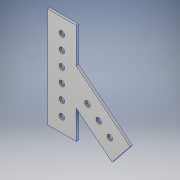
# Autodesk Inventor part: SUP_011_Top4BarBarGusset
Saved by Autodesk Inventor 2018.3 (Build 223284000, 284)
## iProperties
Created: 2020-02-09
Part Number: SUP_011_Top4BarBarGusset
Material: Aluminum 6061
Document SubType Name: Modeling
Designer: 22barlalex
Density: 2.7 g/cm^3
Appearance: Aluminum - Flat
Author: 22barlalex
Autodesk Inventor part; units mm, degrees
ref_plane "YZ Plane" through (0, 0, 0) normal (1, 0, 0) x (0, 1, 0)
ref_plane "XZ Plane" through (0, 0, 0) normal (0, 1, 0) x (-1, 0, 0)
ref_plane "XY Plane" through (0, 0, 0) normal (0, 0, 1) x (1, 0, 0)
sketch "Sketch1" plane through (0, 0, 0) normal (0, 0, 1) x (1, 0, 0)
  line L0 (0, 0) -> (0, 88.9)
  line L1 (0, 88.9) -> (25.4, 88.9)
  line L2 (25.4, 88.9) -> (25.4, 57.9416)
  line L3 (25.4, 57.9416) -> (72.9934, 19.8257)
  line L4 (72.9934, 19.8257) -> (57.1157, 0)
  line L5 (57.1157, 0) -> (25.4, 25.4)
  line L6 (25.4, 25.4) -> (25.4, 0)
  line L7 (25.4, 0) -> (0, 0)
  dimension "d0" = 25.4
  dimension "d1" = 25.4
  dimension "d3" = 25.4
  dimension "d5" = 51.31
  dimension "d18" = 88.9
  constraints: 16 end point, 4 perpendicular, 3 point on line, 1 parallel, 1 vertical
  measures "d0" distance between parallel lines of L3 L5
  measures "d1" distance between parallel lines of L0 L6
  measures "d3" distance of L6.end L5.end
  measures "d5" angle of L5 L6
  measures "d18" distance between parallel lines of L1 L7
extrude "Extrusion1" add sketch "Sketch1" along normal blind 2.032
sketch "Sketch3" plane through (0, 0, 2.032) normal (0, 0, 1) x (1, 0, 0)
  line L0 (25.4, 57.9416) -> (25.4, 88.9) projected
  line L1 (0, 0) -> (25.4, 0) projected
  line L2 (72.9934, 19.8257) -> (25.4, 57.9416) projected
  line L3 (57.1157, 0) -> (72.9934, 19.8257) projected
  point P0 (12.7, 12.7)
  point P1 (12.7, 25.4)
  point P2 (12.7, 38.1)
  point P3 (12.7, 50.8)
  point P4 (12.7, 63.5)
  point P5 (12.7, 76.2)
  point P6 (55.1417, 17.8517)
  point P7 (45.2289, 25.7906)
  point P8 (35.316, 33.7294)
  dimension "d8" = 12.7
  dimension "d9" = 12.7
  dimension "d10" = 12.7
  dimension "d11" = 12.7
  dimension "d12" = 12.7
  dimension "d13" = 12.7
  dimension "d14" = 12.7
  dimension "d19" = 12.7
  dimension "d20" = 12.7
  dimension "d21" = 12.7
  dimension "d23" = 12.7
  dimension "d24" = 12.7
  dimension "d25" = 12.7
  constraints: 5 vertical alignment
  measures "d8" distance from line of L0 point (12.7, 63.5)
  measures "d9" distance from line of L1 point (12.7, 12.7)
  measures "d10" distance of point (12.7, 25.4) point (12.7, 12.7)
  measures "d11" distance of point (12.7, 38.1) point (12.7, 25.4)
  measures "d12" distance of point (12.7, 38.1) point (12.7, 50.8)
  measures "d13" distance of point (12.7, 50.8) point (12.7, 63.5)
  measures "d14" distance of point (12.7, 63.5) point (12.7, 76.2)
  measures "d19" distance from line of L2 point (55.142, 17.852)
  measures "d20" distance from line of L2 point (45.229, 25.791)
  measures "d21" distance from line of L2 point (35.316, 33.729)
  measures "d23" distance from line of L3 point (55.142, 17.852)
  measures "d24" distance of point (55.142, 17.852) point (45.229, 25.791)
  measures "d25" distance of point (45.229, 25.791) point (35.316, 33.729)
hole "Hole1" at (12.7, 12.7, 2.032) at (12.7, 25.4, 2.032) at (12.7, 38.1, 2.032) at (12.7, 50.8, 2.032) at (12.7, 63.5, 2.032) at (12.7, 76.2, 2.032) at (55.1417, 17.8517, 2.032) at (45.2289, 25.7906, 2.032) at (35.316, 33.7294, 2.032) direction (0, 0, -1) diameter 4.8514 end through all
equation "\"d10\" = d9"
equation "\"d11\" = d9"
equation "\"d12\" = d9"
equation "\"d13\" = d9"
equation "\"d14\" = d9"
equation "\"d20\" = d19"
equation "\"d21\" = d19"
equation "\"d23\" = d9"
equation "\"d24\" = d9"
equation "\"d25\" = d9"
body "Solid1"
